Autodesk Inventor part; units mm, degrees
(part 2 of 2)
extrude "Extrusion22" cut sketch "Sketch19" against normal blind 0.4 contours L125 L106 L107 L108 | L108 L107 L106 L125 L114 L113 L112 L126 L127 L128 L129 L130 L116 L117 L118 L121 L122 L123 L124 L110 L111 L109 | L109 L111 L110 L125 | L125 L112 L113 L114 | L114 L41 L112 L125 | L118 L117 L116 L130 | L46 L67 L65 L64 L86 L77 bodies 1
extrude "Extrusion23" add sketch "Sketch19" against normal blind 0.4 contours L125 L106 L107 L108 | L109 L111 L110 L125 | L125 L112 L113 L114 | L114 L41 L112 L125 | L118 L117 L116 L130 | L46 L67 L65 L64 L86 L77 bodies 4
extrude "Extrusion24" add sketch "Sketch19" against normal blind 0.4 contours L125 L106 L107 L108 | L108 L107 L106 L125 L114 L113 L112 L126 L127 L128 L129 L130 L116 L117 L118 L121 L122 L123 L124 L110 L111 L109 | L109 L111 L110 L125 | L125 L112 L113 L114 | L118 L117 L116 L130 bodies 3
extrude "Extrusion25" cut sketch "Sketch19" against normal blind 0.4 contours L125 L106 L107 L108 | L108 L107 L106 L125 L114 L113 L112 L126 L127 L128 L129 L130 L116 L117 L118 L121 L122 L123 L124 L110 L111 L109 | L109 L111 L110 L125 | L125 L112 L113 L114 | L118 L117 L116 L130 bodies 4
